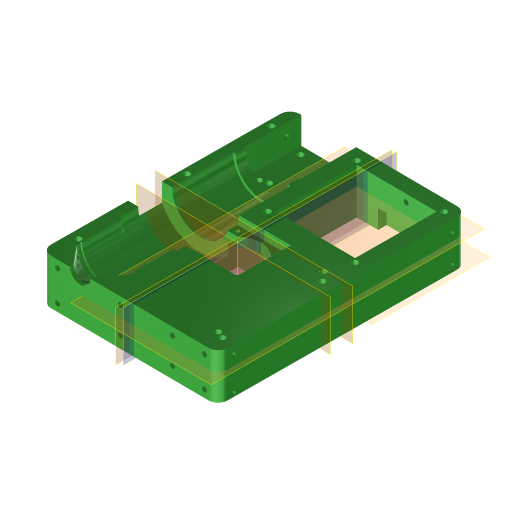
# Autodesk Inventor part: 60_Planktoscope_Base_half_wormdrive_1
Saved by Autodesk Inventor 2024.1 (Build 281209000, 209)
## iProperties
Created: 2024-03-03
Part Number: 60_Planktoscope_Base_half_wormdrive_1
Material: Generisch
Document SubType Name: Modeling
Designer: diederichbenedict
Density: 1 g/cm^3
Appearance: Glatt - Waldgrün
Author: diederichbenedict
Autodesk Inventor part; units mm, degrees
ref_plane "YZ Plane" through (0, 0, 0) normal (1, 0, 0) x (0, 1, 0)
ref_plane "XZ Plane" through (0, 0, 0) normal (0, 1, 0) x (-1, 0, 0)
ref_plane "XY Plane" through (0, 0, 0) normal (0, 0, 1) x (1, 0, 0)
ref_plane "Arbeitsebene1" through (0.1054, 9.1171, 0) normal (0, 0, 1) x (0.9999769, -0.006792, 0)
ref_plane "Arbeitsebene2" through (-59.4, -108.46, 24.3) normal (0, 0, -1) x (0, 1, 0)
sketch "Skizze1" plane through (0.1054, 9.1171, 0) normal (0, 0, 1) x (0.9999769, -0.006792, 0)
  line L0 (19.9723, 13.5324) -> (-22.0277, 13.5324) construction
  line L1 (-22.0277, 13.5324) -> (-22.0277, -28.7676) construction
  line L2 (-22.0277, -28.7676) -> (19.9723, -28.7676) construction
  line L3 (19.9723, -28.7676) -> (19.9723, 13.5324) construction
  line L4 (20.4723, 14.0324) -> (-22.5277, 14.0324)
  line L5 (-22.5277, 14.0324) -> (-22.5277, -29.2676)
  line L6 (-22.5277, -29.2676) -> (20.4723, -29.2676)
  line L7 (20.4723, -29.2676) -> (20.4723, 14.0324)
  circle A0 centre (22.4723, 16.0324) radius 1.4
  circle A1 centre (22.4723, -31.2676) radius 1.4
  circle A2 centre (-24.5277, 16.0324) radius 1.4
  circle A3 centre (-24.5277, -31.2676) radius 1.4
  line L8 (28.4723, 22.0324) -> (-66.5277, 22.0324) construction
  line L9 (-66.5277, 22.0324) -> (-66.5277, -109.9676) construction
  line L10 (-66.5277, -109.9676) -> (28.4723, -109.9676) construction
  line L11 (28.4723, -109.9676) -> (28.4723, 22.0324) construction
  line L12 (28.4723, 22.0324) -> (-66.5277, 22.0324)
  line L13 (-66.5277, 22.0324) -> (-66.5277, -109.9676)
  line L14 (-66.5277, -109.9676) -> (28.4723, -109.9676)
  line L15 (28.4723, -109.9676) -> (28.4723, 22.0324)
  line L16 (-2.5256, -40.7176) -> (-31.0256, -40.7176)
  line L17 (-31.0256, -40.7176) -> (-31.0256, -69.2176)
  line L18 (-31.0256, -69.2176) -> (-2.5256, -69.2176)
  line L19 (-2.5256, -69.2176) -> (-2.5256, -40.7176)
  line L20 (-2.5256, -40.7176) -> (-31.0256, -69.2176)
  line L21 (-31.0256, -40.7176) -> (-2.5256, -69.2176)
  line L22 (-45.6017, -54.4502) -> (-45.6221, -39.4502) construction
  point P0 (-0.0435, -9.1176)
  point P1 (-16.7756, -54.9676)
  dimension "d0" = 0.5
  dimension "d1" = 2.8
  dimension "d2" = 2.8
  dimension "d3" = 2.8
  dimension "d4" = 2.8
  dimension "d5" = 95
  dimension "d6" = 132
  dimension "d41" = 31.15
  dimension "d92" = 28.5
  dimension "d93" = 28.5
  dimension "d105" = 55
  dimension "d107" = 43.3
  dimension "d108" = 43
  dimension "d109" = 2
  dimension "d110" = 2
  dimension "d111" = 2
  dimension "d112" = 2
  dimension "d113" = 2
  dimension "d114" = 2
  dimension "d115" = 2
  dimension "d116" = 2
  dimension "d117" = 8
  dimension "d118" = 8
  constraints: 46 end point, 10 parallel, 5 perpendicular, 4 centre point, 4 horizontal, 2 midpoint, 3 other
  measures "d0" distance between parallel lines of L3 L7
  measures "d1" diameter of A0
  measures "d2" diameter of A1
  measures "d3" diameter of A2
  measures "d4" diameter of A3
  measures "d5" distance of L10.end L9.end
  measures "d6" distance of L9.end L8.end
  measures "d41" distance from line of L8 point (-0.043, -9.118)
  measures "d92" distance of L18.end L17.end
  measures "d93" distance of L17.end L16.end
  measures "d105" distance from line of point (-16.776, -54.968) L10
  measures "d107" distance between parallel lines of L4 L6
  measures "d108" distance between parallel lines of L5 L7
  measures "d109" distance from line of L7 A1.centre
  measures "d110" distance from line of L7 A0.centre
  measures "d111" distance from line of L4 A0.centre
  measures "d112" distance from line of L6 A1.centre
  measures "d113" distance from line of L6 A3.centre
  measures "d114" distance from line of A3.centre L5
  measures "d115" distance from line of A2.centre L5
  measures "d116" distance from line of A2.centre L4
  measures "d117" distance between parallel lines of L8 L4
  measures "d118" distance between parallel lines of L11 L7
extrude "Extrusion1" add sketch "Skizze1" along normal up to surface (24.3 mm away)
sketch "Skizze2" plane through (-66.2711, 31.6008, 24.3) normal (0, 0, 1) x (0.9999769, -0.006792, 0)
  line L0 (44, -8) -> (87, -8) projected
  line L1 (87, -8) -> (87, -51.3) projected
  line L2 (87, -51.3) -> (44, -51.3) projected
  line L3 (44, -51.3) -> (44, -8) projected
  circle A0 centre (89, -53.3) radius 1.4 projected
  circle A1 centre (42, -53.3) radius 1.4 projected
  line L4 (95, 0) -> (0, 0) projected
  line L5 (0, 0) -> (0, -132) projected
  line L6 (0, -132) -> (95, -132) projected
  line L7 (95, -132) -> (95, 0) projected
  line L8 (7.35, -118.91) -> (7.35, -120.06)
  arc A2 (7.35, -118.91) -> (7.35, -117.91) centre (7.35, -118.41) ccw construction
  line L9 (7.35, -96.06) -> (7.35, -117.91) construction
  line L10 (7.35, -85.56) -> (7.35, -94.56)
  line L11 (6.25, -70.56) -> (6.25, -85.56)
  line L12 (6.25, -35.3731) -> (6.25, -70.06)
  line L13 (20.85, -132) -> (20.85, 0) construction
  line L14 (15.35, -128.06) -> (15.35, -132)
  line L15 (7.35, -96.06) -> (7.35, -94.56)
  line L16 (7.35, -85.56) -> (6.25, -85.56)
  line L17 (6.25, -70.56) -> (6.25, -70.06)
  line L18 (15.1, -132) -> (15.1, -128.1636)
  line L19 (7.1, -120.1636) -> (7.1, -118.41)
  arc A3 (7.1, -118.41) -> (7.1, -118.41) centre (7.35, -118.41) ccw
  line L20 (7.1, -118.41) -> (7.1, -96.0507)
  line L21 (7.1, -96.0507) -> (7.1, -94.56)
  line L22 (7.1, -94.56) -> (7.1, -85.81)
  line L23 (7.1, -85.81) -> (6, -85.81)
  line L24 (6, -85.81) -> (6, -70.56)
  line L25 (6, -70.56) -> (6, -70.06)
  line L26 (6, -70.06) -> (6, -35.6231)
  line L27 (6, -35.6231) -> (35.4785, -35.6231)
  line L28 (6.8285, -35.6231) -> (6.8285, -21.377)
  line L29 (6.8285, -21.377) -> (20.85, -21.377)
  line L30 (20.85, -21.377) -> (20.85, -132)
  line L31 (15.1, -132) -> (20.85, -132)
  line L32 (7.1, -97.4127) -> (7.2407, -96.0654)
  line L33 (7.2407, -96.0654) -> (7.1, -96.0507)
  circle A4 centre (7.1, -117.9136) radius 0.5
  line L34 (7.35, -120.06) -> (15.35, -129.594) construction
  line L35 (15.35, -130.03) -> (7.1, -120.198)
  line L36 (7.1, -120.198) -> (7.1, -120.1636)
  line L37 (20.85, -35.6231) -> (5.45, -35.6231)
  line L38 (5.45, -35.6231) -> (5.45, -85.81)
  line L39 (5.45, -85.81) -> (20.85, -85.81)
  line L40 (20.85, -85.81) -> (20.85, -35.6231)
  line L41 (20.85, -85.81) -> (5.45, -85.81)
  line L42 (5.45, -85.81) -> (5.45, -96.0654)
  line L43 (5.45, -96.0654) -> (20.85, -96.0654)
  line L44 (20.85, -96.0654) -> (20.85, -85.81)
  point P0 (66.4842, -31.15)
  point P1 (6.2644, -35.3731)
  point P2 (7.1, -118.4136)
  point P3 (7.1, -117.4136)
  point P4 (15.1, -129.7321)
  point P5 (6, -35.6231)
  point P6 (6, -85.81)
  point P7 (6, -85.81)
  point P8 (5.45, -85.81)
  point P9 (7.1, -96.0654)
  dimension "d9" = 0.25
  dimension "d74" = 1
  dimension "d75" = 2.25
  dimension "d104" = 15.4
  constraints: 74 end point, 9 point on line, 9 vertical, 7 perpendicular, 5 parallel, 4 point on circle, 3 centre point, 3 horizontal, 2 collinear, 1 midpoint, 22 other
  measures "d9" distance between parallel lines of L9 L20
  measures "d74" diameter of A4
  measures "d75" distance of A4.centre L19.start
  measures "d104" distance of L39.end L38.end
revolve "Umdrehung1" cut sketch "Skizze2" angle 360 about axis through (-46.3181, -100.5377, 24.3) along (0.006792, 0.9999769, 0) contours L6 L14 L35 L36 L19 A3 A4 L20 L32 L43 L30 | L43 L33 L21 L22 L39 L30 | L39 L10 L16 L11 L17 L12 L27 L30 | L27 L28 L29 L30 | L39 L23 L24 L25 L26 L27 L12 L17 L11 L16 L10 | L20 L43 L42 L39 L23 L22 L21 | A4 A3 L20 | L20 L19 A4 | A4 A3 | L19 A3 A4 | L39 L38 L37 L26 L25 L24
sketch "Skizze5" plane through (-66.2711, 31.6008, 24.3) normal (0, 0, 1) x (0.9999769, -0.006792, 0)
  line L0 (26.35, -132) -> (95, -132) projected
  line L1 (95, -132) -> (95, 0) projected
  line L2 (44, -8) -> (87, -8) projected
  line L3 (87, -8) -> (87, -51.3) projected
  line L4 (87, -51.3) -> (44, -51.3) projected
  line L5 (44, -51.3) -> (44, -8) projected
  circle A0 centre (89, -53.3) radius 1.4 projected
  circle A1 centre (42, -53.3) radius 1.4 projected
  line L6 (35.3118, 7.597) -> (35.3464, -17.9029) projected
  line L7 (6.3465, -17.942) -> (6.3118, 7.5576) projected
  line L8 (35.35, -30.064) -> (6.2848, -30.064)
  line L9 (6.2848, -30.064) -> (6.2848, 0)
  line L10 (6.2848, 0) -> (35.35, 0)
  line L11 (35.35, 0) -> (35.35, -30.064)
  line L12 (35.65, -30.364) -> (5.9848, -30.364)
  line L13 (5.9848, -30.364) -> (5.9848, 0.3)
  line L14 (5.9848, 0.3) -> (35.65, 0.3)
  line L15 (35.65, 0.3) -> (35.65, -30.364)
  line L16 (0, 0) -> (0, -132) projected
  line L17 (34.6, -96.0507) -> (34.4593, -96.0654) projected
  line L18 (34.4593, -96.0654) -> (34.6, -97.4127) projected
  line L19 (34.6, -97.4127) -> (34.6, -117.4136) projected
  arc A2 (34.6, -118.4136) -> (34.6, -117.4136) centre (34.6, -117.9136) ccw projected
  line L20 (34.6, -118.4136) -> (34.6, -120.198) projected
  line L21 (34.6, -120.198) -> (26.35, -130.03) projected
  line L22 (26.35, -130.03) -> (26.35, -132) projected
  line L23 (6.8285, -35.6231) -> (6.8285, -21.377) projected
  line L24 (6.8285, -21.377) -> (34.8715, -21.377) projected
  line L25 (34.8715, -21.377) -> (34.8715, -35.6231) projected
  line L26 (0, -132) -> (15.35, -132) projected
  line L27 (15.35, -132) -> (15.35, -130.03) projected
  line L28 (15.35, -130.03) -> (7.1, -120.198) projected
  line L29 (7.1, -120.198) -> (7.1, -118.4136) projected
  arc A3 (7.1, -117.4136) -> (7.1, -118.4136) centre (7.1, -117.9136) ccw projected
  line L30 (7.1, -117.4136) -> (7.1, -97.4127) projected
  line L31 (7.1, -97.4127) -> (7.2407, -96.0654) projected
  line L32 (7.2407, -96.0654) -> (7.1, -96.0507) projected
  line L33 (64.002, -91.25) -> (36.25, -91.25) projected
  line L34 (36.25, -62.75) -> (64.002, -62.75) projected
  line L35 (64.002, -62.75) -> (64.002, -91.25) projected
  line L36 (95, 0) -> (0, 0) projected
  line L37 (36.25, -35.6231) -> (36.25, -62.75) projected
  line L38 (5.45, -35.6231) -> (6.8285, -35.6231) projected
  line L39 (34.8715, -35.6231) -> (36.25, -35.6231) projected
  line L40 (36.25, -91.25) -> (36.25, -96.0654) projected
  line L41 (36.25, -96.0654) -> (34.6, -96.0654) projected
  line L42 (34.6, -96.0654) -> (34.6, -96.0507) projected
  line L43 (7.1, -96.0507) -> (7.1, -96.0654) projected
  line L44 (7.1, -96.0654) -> (5.45, -96.0654) projected
  line L45 (5.45, -96.0654) -> (5.45, -35.6231) projected
  point P0 (66.4842, -31.15)
  point P1 (26.2848, -132)
  dimension "d23" = 0.3
  constraints: 16 end point, 4 parallel, 2 perpendicular, 1 horizontal, 3 other
  measures "d23" distance between parallel lines of L11 L15
extrude "Extrusion4" cut sketch "Skizze5" against normal blind 14.3 contours L36 L10 L6 L14 L15 | L15 L12 L25 L8 L11 L36 | L11 L8 L25 L24 L23 L9 L10 | L6 L10 L7 L14 | L12 L23 L8 L25 | L7 L10 L36 L13 L14 | L12 L13 L36 L9 L8 L23 | L8 L23 L24 L25
sketch "Skizze6" plane through (0.1054, 9.1171, 0) normal (0, 0, -1) x (-0.9999769, 0.006792, 0)
  line L0 (66.5277, 22.0324) -> (66.5277, -109.9676) construction
  line L1 (-28.4723, 22.0324) -> (66.5277, 22.0324) construction
  line L2 (-28.4723, -109.9676) -> (-28.4723, 22.0324) construction
  line L3 (66.5277, -109.9676) -> (-28.4723, -109.9676) construction
  circle A0 centre (24.5277, -31.2676) radius 1.4 projected
  circle A1 centre (-22.4723, -31.2676) radius 1.4 projected
  line L4 (-20.4723, 14.0324) -> (-20.4723, -29.2676) projected
  line L5 (22.5277, 14.0324) -> (-20.4723, 14.0324) projected
  line L6 (22.5277, -29.2676) -> (22.5277, 14.0324) projected
  line L7 (-20.4723, -29.2676) -> (22.5277, -29.2676) projected
  line L8 (-18.4723, -99.9676) -> (-18.4723, 12.0324) construction
  line L9 (-18.4723, 12.0324) -> (56.5277, 12.0324) construction
  line L10 (56.5277, 12.0324) -> (56.5277, -99.9676) construction
  line L11 (56.5277, -99.9676) -> (-18.4723, -99.9676) construction
  circle A2 centre (-22.4723, 16.0324) radius 1.4 projected
  circle A3 centre (24.5277, 16.0324) radius 1.4 projected
  point P0 (0.0435, -9.1176)
  point P1 (-18.4723, -43.9676)
  point P2 (-22.5409, -48.7573)
  point P3 (-22.3224, -101.5013)
  point P4 (63.2779, 8.8575)
  point P5 (63.3848, -35.7623)
  point P6 (61.8771, -94.8224)
  dimension "d26" = 10
  constraints: 8 end point, 3 coincident, 1 midpoint, 3 other
  measures "d26" distance between parallel lines of L3 L11
hole "Bohrung1" at (17.8983, -90.9737, 0) at (18.2787, -34.975, 0) at (22.3146, -39.7922, 0) at (21.738, -92.5334, 0) at (-63.5208, -26.2138, 0) at (-63.1109, 18.4042, 0) at (-62.4142, -85.2828, 0) at (22.3649, -22.3024, 0) at (22.6861, 24.9965, 0) at (-24.3128, 25.3157, 0) at (-24.6341, -21.9832, 0) direction (0, 0, 1) diameter 3.3 end through all counterbore diameter 4 counterbore depth 8
sketch "Skizze8" plane through (-45.6479, -100.5423, 24.3) normal (-0.006792, -0.9999769, 0) x (0.9999769, -0.006792, 0)
  line L0 (-21.5202, 0) -> (-6.1702, 0) projected
  line L1 (4.8298, 0) -> (73.4798, 0) projected
  line L2 (-21.5202, -24.3) -> (73.4798, -24.3) projected
  line L3 (66.15, -20.3) -> (66.15, -4) construction
  line L4 (66.15, -4) -> (48.9999, -4) construction
  line L5 (48.9999, -4) -> (48.9999, -18.1) construction
  line L6 (48.9999, -18.1) -> (20.9999, -18.1) construction
  line L7 (20.9999, -18.1) -> (20.9999, -4) construction
  line L8 (20.9999, -4) -> (8.8917, -4) construction
  arc A0 (-8.8917, -4) -> (8.8917, -4) centre (0, 0) ccw construction
  line L9 (-8.8917, -4) -> (-12.85, -4) construction
  line L10 (-12.85, -4) -> (-12.85, -20.3) construction
  line L11 (-12.85, -20.3) -> (66.15, -20.3) construction
  line L12 (-21.5202, -24.3) -> (-21.5202, 0) projected
  line L13 (73.4798, -24.3) -> (73.4798, 0) projected
  arc A1 (-6.1702, 0) -> (4.8298, 0) centre (-0.6702, 0) ccw projected
  point P0 (44.964, -24.3)
  point P1 (5.2944, 0)
  point P2 (73.9444, 0)
  constraints: 18 end point, 8 coincident, 2 point on circle, 1 centre point
hole "Bohrung2" at (20.5006, -100.9916, 4) at (20.5006, -100.9916, 20.3) at (3.3508, -100.8751, 6.2) at (-24.6485, -100.6849, 6.2) at (-24.6485, -100.6849, 20.3) at (-58.4976, -100.455, 20.3) at (3.3508, -100.8751, 20.3) at (-58.4976, -100.455, 4) direction (0.006792, 0.9999769, 0) diameter 2.8 depth 12 tip angle 118
sketch "Skizze13" plane through (0.1054, 9.1171, 0) normal (0, 0, -1) x (-0.9999769, 0.006792, 0)
  line L0 (-20.4723, 14.0324) -> (-20.4723, -29.2676) projected
  line L1 (22.5277, 14.0324) -> (-20.4723, 14.0324) projected
  line L2 (22.5277, -29.2676) -> (22.5277, 14.0324) projected
  line L3 (-20.4723, -29.2676) -> (22.5277, -29.2676) projected
  line L4 (-28.4723, -109.9676) -> (-28.4723, 22.0324) projected
  line L5 (66.5277, -109.9676) -> (-28.4723, -109.9676) projected
  line L6 (66.5277, 22.0324) -> (66.5277, -109.9676) projected
  line L7 (-28.4723, 22.0324) -> (66.5277, 22.0324) projected
  line L8 (11.0277, 9.5324) -> (-8.9723, 9.5324)
  line L9 (-8.9723, 9.5324) -> (-8.9723, 18.5324)
  line L10 (-8.9723, 18.5324) -> (11.0277, 18.5324)
  line L11 (11.0277, 18.5324) -> (11.0277, 9.5324)
  line L12 (11.0277, 9.5324) -> (-8.9723, 18.5324) construction
  line L13 (-8.9723, 9.5324) -> (11.0277, 18.5324) construction
  point P0 (0.0435, -9.1176)
  point P1 (1.0277, 14.0324)
  dimension "d80" = 20
  dimension "d81" = 9
  constraints: 12 end point, 3 midpoint, 2 parallel, 1 horizontal, 1 perpendicular
  measures "d80" distance of L9.end L10.end
  measures "d81" distance of L8.end L9.end
extrude "Extrusion7" cut sketch "Skizze13" against normal blind 10 contours L9 L10 L11 L1 | L1 L11 L8 L9
fillet "Rundung2" radius 5 4 edges at (27.8302, -101.0414, 12.15) (-67.1676, -100.3961, 12.15) (28.7267, 30.9556, 12.15) (-66.2711, 31.6008, 12.15)
sketch "Skizze14" plane through (27.8641, -96.0415, 0) normal (0.9999769, -0.006792, 0) x (0, 0, -1)
  line L0 (-19.3, 3) -> (-3, 3)
  line L1 (-3, 3) -> (-3, 119)
  line L2 (-3, 119) -> (-19.3, 119)
  line L3 (-19.3, 119) -> (-19.3, 3)
  line L4 (-24.3, 0) -> (-24.3, 122) projected
  point P0 (0, 95.85)
  point P1 (-17.748, 119)
  point P2 (-1.448, 3)
  dimension "d119" = 16.3
  dimension "d120" = 116
  dimension "d121" = 5
  constraints: 8 end point, 2 parallel, 1 horizontal, 1 perpendicular
  measures "d119" distance between parallel lines of L1 L3
  measures "d120" distance between parallel lines of L2 L0
  measures "d121" distance between parallel lines of L4 L3
hole "Bohrung6" at (28.6724, 22.9558, 3) at (28.6724, 22.9558, 17.748) at (27.8845, -93.0415, 1.448) at (27.8845, -93.0415, 19.3) direction (-0.9999769, 0.006792, 0) diameter 2.8 depth 12 tip angle 118
ref_plane "Arbeitsebene3" through (-31.2929, -45.6385, 0) normal (-0.006792, -0.9999769, 0) x (0.9999769, -0.006792, 0)
ref_plane "Arbeitsebene4" through (-17.14, -59.985, 0) normal (-0.9999769, 0.006792, 0) x (0, 0, 1)
ref_plane "Arbeitsebene5" through (-31.1961, -31.3888, 14.3) normal (0, 0, 1) x (0.9999769, -0.006792, 0)
sketch "Skizze15" plane through (-31.1961, -31.3888, 14.3) normal (0, 0, 1) x (0.9999769, -0.006792, 0)
  circle A0 centre (25.7344, -2.7344) radius 1.9 projected
  circle A1 centre (25.7656, -25.7344) radius 1.9 projected
  circle A2 centre (2.7656, -25.7656) radius 1.9 projected
  circle A3 centre (2.7344, -2.7656) radius 1.9 projected
  circle A4 centre (14.25, -14.25) radius 3.75 projected
  circle A5 centre (14.25, -14.25) radius 10.8 projected
  circle A6 centre (14.25, -14.25) radius 12.5
  circle A7 centre (53.3481, -60.7837) radius 1.65 projected
  circle A8 centre (53.5665, -8.0397) radius 1.65 projected
  circle A9 centre (49.498, -3.25) radius 1.65 projected
  circle A10 centre (49.498, -59.25) radius 1.65 projected
  line L0 (8.498, 54.75) -> (51.498, 54.75) projected
  line L1 (51.498, 54.75) -> (51.498, 11.45) projected
  line L2 (51.498, 11.45) -> (8.498, 11.45) projected
  line L3 (8.498, 11.45) -> (8.498, 54.75) projected
  line L4 (54.498, 62.75) -> (0.148, 62.75) projected
  line L5 (0.148, 62.75) -> (0.148, 32.386) projected
  line L6 (0.148, 32.386) -> (-0.6305, 32.386) projected
  line L7 (-0.6305, 32.386) -> (-0.6305, 27.1269) projected
  line L8 (0.748, 0) -> (28.5, 0) projected
  line L9 (28.5, 0) -> (28.5, -28.5) projected
  line L10 (28.5, -28.5) -> (0.748, -28.5) projected
  line L11 (-0.902, -33.3007) -> (-1.0427, -33.3154) projected
  line L12 (-1.0427, -33.3154) -> (-0.902, -34.6627) projected
  line L13 (-0.902, -34.6627) -> (-0.902, -54.6636) projected
  arc A11 (-0.902, -55.6636) -> (-0.902, -54.6636) centre (-0.902, -55.1636) ccw projected
  line L14 (-0.902, -55.6636) -> (-0.902, -57.448) projected
  line L15 (-0.902, -57.448) -> (-9.152, -67.28) projected
  line L16 (-9.152, -67.28) -> (-9.152, -69.25) projected
  line L17 (-9.152, -69.25) -> (54.498, -69.25) projected
  line L18 (59.498, -64.25) -> (59.498, 57.75) projected
  line L19 (28.5, 0) -> (0, 0)
  line L20 (0, 0) -> (0, -28.496)
  line L21 (0, -28.496) -> (28.5, -28.496)
  line L22 (28.5, -28.496) -> (28.5, 0)
  circle A12 centre (25.7344, -2.7344) radius 1.025 projected
  circle A13 centre (25.7656, -25.7344) radius 1.025 projected
  circle A14 centre (2.7344, -2.7656) radius 1.025 projected
  circle A15 centre (2.7656, -25.7656) radius 1.025 projected
  line L23 (-35.502, 57.75) -> (-35.502, -64.25) projected
  line L24 (-30.502, -69.25) -> (-20.152, -69.25) projected
  line L25 (-20.152, -69.25) -> (-20.152, -67.28) projected
  line L26 (-20.152, -67.28) -> (-28.402, -57.448) projected
  line L27 (-28.402, -57.448) -> (-28.402, -55.6636) projected
  arc A16 (-28.402, -54.6636) -> (-28.402, -55.6636) centre (-28.402, -55.1636) ccw projected
  line L28 (-28.402, -54.6636) -> (-28.402, -34.6627) projected
  line L29 (-28.402, -34.6627) -> (-28.2614, -33.3154) projected
  line L30 (-28.2614, -33.3154) -> (-28.402, -33.3007) projected
  line L31 (-29.5172, 62.75) -> (-30.502, 62.75) projected
  line L32 (-28.6735, 27.1269) -> (-28.6735, 32.386) projected
  line L33 (-28.6735, 32.386) -> (-29.5172, 32.386) projected
  arc A17 (-35.502, -64.25) -> (-30.502, -69.25) centre (-30.502, -64.25) ccw projected
  arc A18 (59.498, 57.75) -> (54.498, 62.75) centre (54.498, 57.75) ccw projected
  arc A19 (54.498, -69.25) -> (59.498, -64.25) centre (54.498, -64.25) ccw projected
  line L34 (-0.6305, 27.1269) -> (0.748, 27.1269) projected
  line L35 (0.748, 27.1269) -> (0.748, 0) projected
  line L36 (-30.052, 27.1269) -> (-28.6735, 27.1269) projected
  circle A20 centre (-30.8514, -54.1048) radius 1.65 projected
  circle A21 centre (-32.3591, 4.9553) radius 1.65 projected
  circle A22 centre (-32.2523, 49.5751) radius 1.65 projected
  line L37 (-29.5172, 32.386) -> (-29.5172, 62.75) projected
  arc A23 (-30.502, 62.75) -> (-35.502, 57.75) centre (-30.502, 57.75) ccw projected
  line L38 (0.748, -28.5) -> (0.748, -33.3154) projected
  line L39 (0.748, -33.3154) -> (-0.902, -33.3154) projected
  line L40 (-0.902, -33.3154) -> (-0.902, -33.3007) projected
  line L41 (-28.402, -33.3007) -> (-28.402, -33.3154) projected
  line L42 (-28.402, -33.3154) -> (-30.052, -33.3154) projected
  line L43 (-30.052, -33.3154) -> (-30.052, 27.1269) projected
  point P0 (30.9822, 31.6)
  point P1 (-9.8862, -78.2185)
  point P2 (27.5984, -28.496)
  point P3 (28.5, -28.496)
  point P4 (0.9022, -28.496)
  dimension "d97" = 25
  constraints: 8 end point, 2 parallel, 1 centre point, 1 coincident, 1 horizontal, 1 perpendicular
  measures "d97" diameter of A6
extrude "Extrusion8" add sketch "Skizze15" along normal blind 5 contours A0 | A1 | A2 | A3 | L8 L9 L21 L20 L19
sketch "Skizze16" plane through (-31.2929, -45.6385, 0) normal (-0.006792, -0.9999769, 0) x (0.9999769, -0.006792, 0)
  ellipse E0 centre (-15.3031, 24.3) end of major axis (-15.3031, 10.8) minor radius 13.5 projected
  circle A0 centre (-15.3031, 24.3) radius 22.5
  point P0 (30.9822, 0)
  dimension "d101" = 45
  constraints: 1 centre point, 1 coincident
  measures "d101" diameter of A0
extrude "Extrusion9" cut sketch "Skizze16" along normal mid plane 18 contours E0 | A0
ref_plane "Arbeitsebene6" through (-18.8061, 26.2783, 24.3) normal (0.9999769, -0.006792, 0) x (0, 0, -1)
mirror "Spiegeln1" about plane through (-18.8061, 26.2783, 24.3) normal (0.9999769, -0.006792, 0) of "Bohrung6"
ref_plane "Arbeitsebene7" through (-61.7195, -34.4316, 0) normal (-0.006792, -0.9999769, 0) x (0.9999769, -0.006792, 0)
mirror "Spiegeln2" about plane through (-61.7195, -34.4316, 0) normal (-0.006792, -0.9999769, 0) of "Bohrung2"
sketch "Skizze17" plane through (0.1054, 9.1171, 0) normal (0, 0, -1) x (-0.9999769, 0.006792, 0)
  circle A0 centre (35.6777, -5.2176) radius 1.25 projected
  arc A1 (56.2581, 20.2824) -> (53.7561, 17.8042) centre (56.256, 17.7824) ccw projected
  line L0 (58.9699, 20.2827) -> (56.2581, 20.2825) projected
  line L1 (58.9699, 20.2827) -> (58.9703, -7.2187) projected
  spline S0 degree 3 poles (58.0783, -7.9028) (58.1331, -7.8973) (58.1875, -7.8879) (58.2425, -7.8745) (58.2975, -7.861) (58.3531, -7.8436) (58.4059, -7.8233) (58.4587, -7.803) (58.5085, -7.7799) (58.5536, -7.7559) (58.5986, -7.7318) (58.639, -7.7068) (58.6754, -7.6812) (58.7118, -7.6556) (58.7444, -7.6294) (58.7735, -7.6029) (58.8025, -7.5763) (58.8281, -7.5493) (58.8502, -7.5224) (58.8723, -7.4955) (58.8909, -7.4686) (58.9064, -7.4421) (58.9218, -7.4157) (58.934, -7.3896) (58.9435, -7.3643) (58.953, -7.339) (58.9598, -7.3144) (58.9641, -7.2899) (58.9684, -7.2653) (58.9703, -7.2408) (58.9703, -7.2187) knots 0 0 0 0 0.1 0.1 0.1 0.2 0.2 0.2 0.3 0.3 0.3 0.4 0.4 0.4 0.5 0.5 0.5 0.6 0.6 0.6 0.7 0.7 0.7 0.8 0.8 0.8 0.9 0.9 0.9 1 1 1 1 projected
  spline S1 degree 3 poles (33.2771, -7.9028) (33.3794, -7.9132) (33.5968, -7.9192) (33.9386, -7.9172) (34.3134, -7.9178) (34.7222, -7.9176) (35.168, -7.9177) (35.6549, -7.9176) (36.1877, -7.9176) (36.772, -7.9176) (37.4141, -7.9176) (38.1218, -7.9176) (38.9042, -7.9176) (39.773, -7.9176) (40.7418, -7.9176) (41.8297, -7.9176) (43.0552, -7.9176) (44.3904, -7.9176) (45.7546, -7.9176) (47.0654, -7.9176) (48.2835, -7.9176) (49.4158, -7.9176) (50.4682, -7.9176) (51.4464, -7.9176) (52.3555, -7.9176) (53.2003, -7.9176) (53.9852, -7.9176) (54.7142, -7.9176) (55.3908, -7.9176) (56.018, -7.9176) (56.5982, -7.9176) (57.1328, -7.9176) (57.6209, -7.9177) (57.9321, -7.9175) (58.0783, -7.9028) knots 0 0 0 0 0.012454 0.026265 0.041356 0.057789 0.075708 0.095278 0.116688 0.140158 0.165945 0.194355 0.225757 0.26059 0.299437 0.342945 0.392182 0.44767 0.504448 0.55719 0.606219 0.651791 0.694148 0.733518 0.770107 0.804111 0.835704 0.865049 0.892289 0.917546 0.940917 0.962464 0.982201 1 1 1 1 projected
  spline S2 degree 3 poles (32.3848, -7.2198) (32.3849, -7.2353) (32.3869, -7.2674) (32.3958, -7.3158) (32.4111, -7.3652) (32.433, -7.4149) (32.4617, -7.4647) (32.4978, -7.5148) (32.5417, -7.5651) (32.5943, -7.6154) (32.6566, -7.6658) (32.7299, -7.7158) (32.8157, -7.7648) (32.9158, -7.8117) (33.0296, -7.8534) (33.1516, -7.8854) (33.2357, -7.8986) (33.2771, -7.9028) knots 0.000644 0.000644 0.000644 0.000644 0.046478 0.094952 0.144249 0.194804 0.247064 0.301535 0.358802 0.419552 0.484614 0.554981 0.631878 0.716385 0.809647 0.906987 1 1 1 1 projected
  line L2 (32.3851, -7.2191) -> (32.3855, 20.2827) projected
  line L3 (32.3855, 20.2827) -> (35.0978, 20.2825) projected
  arc A2 (37.5993, 17.8042) -> (35.0978, 20.2824) centre (35.0994, 17.7824) ccw projected
  line L4 (37.6048, 17.171) -> (37.5993, 17.8042) projected
  arc A3 (37.6048, 17.171) -> (38.9048, 15.8824) centre (38.9048, 17.1824) ccw projected
  line L5 (52.4506, 15.8824) -> (38.9048, 15.8824) projected
  arc A4 (52.4506, 15.8824) -> (53.7505, 17.171) centre (52.4506, 17.1824) ccw projected
  line L6 (53.7505, 17.171) -> (53.7561, 17.8042) projected
  circle A5 centre (34.6777, 17.7824) radius 1.6 projected
  line L7 (32.9777, 14.8324) -> (55.7777, 14.8324) projected
  line L8 (32.9777, -0.5676) -> (32.9777, 14.8324) projected
  line L9 (58.3777, -0.5676) -> (32.9777, -0.5676) projected
  line L10 (58.3777, 11.8324) -> (58.3777, -0.5676) projected
  line L11 (55.7777, 14.8324) -> (58.3777, 11.8324) projected
  circle A6 centre (35.6777, -5.2176) radius 1.55 projected
  circle A7 centre (39.6777, -3.7176) radius 1.1 projected
  circle A8 centre (51.6777, -3.7176) radius 1.1 projected
  circle A9 centre (55.6777, -5.2176) radius 1.55 projected
  circle A10 centre (56.6777, 17.7824) radius 1.6 projected
  point P0 (0.0435, -9.1176)
hole "Bohrung7" at (-55.6064, 4.2778, 0) at (-35.6069, 4.1419, 0) at (-56.4502, 27.284, 0) at (-34.8724, 27.1375, 0) at (-34.4507, 27.1346, 0) at (-51.5963, 5.7506, 0) at (-39.5966, 5.6691, 0) direction (0, 0, 1) diameter 3.3 end through all counterbore diameter 7 counterbore depth 3
